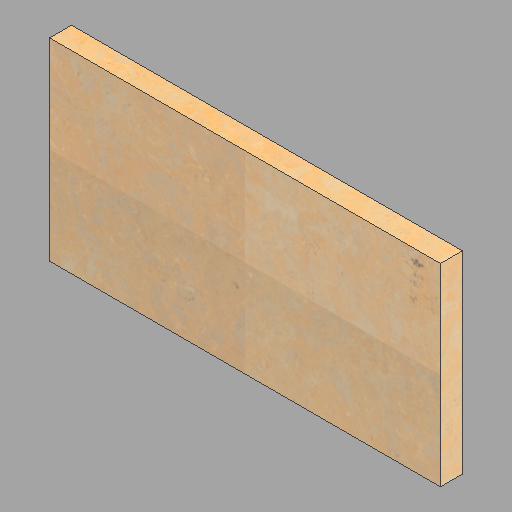
# Autodesk Inventor part: 10 - panel - 214
Saved by Autodesk Inventor 2023 (Build 270158000, 158)
## iProperties
RuleStatus: InUse
Created: 2022-03-21
Part Number: 10 - panel - 214
Material: Granite, Cut, Polished
Document SubType Name: Modeling
Designer: awelt
Mass: 55562.1 g
Surface Area: 9475.99 cm^2
Volume: 20578.6 cm^3
Density: 2.7 g/cm^3
Appearance: Amber Select
AfterDocSave0: Convert in3 volume to ft3
in3 to ft3: 0.73
TEST: 0.727
Author: awelt
Autodesk Inventor part; units mm, degrees
ref_plane "YZ Plane" through (0, 0, 0) normal (1, 0, 0) x (0, 1, 0)
ref_plane "XZ Plane" through (0, 0, 0) normal (0, 1, 0) x (-1, 0, 0)
ref_plane "XY Plane" through (0, 0, 0) normal (0, 0, 1) x (1, 0, 0)
sketch "Sketch1" plane through (0, 0, 0) normal (0, 0, 1) x (1, 0, 0)
  line L0 (-452.4375, 223.8375) -> (452.4375, 223.8375)
  line L1 (452.4375, 223.8375) -> (452.4375, -223.8375)
  line L2 (452.4375, -223.8375) -> (-452.4375, -223.8375)
  line L3 (-452.4375, -223.8375) -> (-452.4375, 223.8375)
  line L4 (-452.4375, 223.8375) -> (452.4375, -223.8375) construction
  line L5 (452.4375, 223.8375) -> (-452.4375, -223.8375) construction
  point P0 (0, 0)
  dimension "d0" = 904.875
  dimension "d1" = 447.675
  constraints: 12 end point, 2 midpoint, 2 parallel, 1 horizontal, 1 perpendicular
  measures "d0" distance of L1.end L2.end
  measures "d1" distance of L0.end L1.end
extrude "Extrusion1" add sketch "Sketch1" along normal blind 50.8
body "Solid1"
